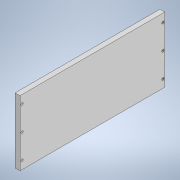
# Autodesk Inventor part: cab_L_L
Saved by Autodesk Inventor 2022 (Build 260153000, 153)
## iProperties
Created: 2023-03-05
Part Number: cab_L_L
Material: Generic
Document SubType Name: Modeling
Designer: Bunny
Density: 1 g/cm^3
Appearance: Default
Author: Bunny
Autodesk Inventor part; units mm, degrees
ref_plane "YZ Plane" through (0, 0, 0) normal (1, 0, 0) x (0, 1, 0)
ref_plane "XZ Plane" through (0, 0, 0) normal (0, 1, 0) x (-1, 0, 0)
ref_plane "XY Plane" through (0, 0, 0) normal (0, 0, 1) x (1, 0, 0)
sketch "Sketch1" plane through (0, 0, 0) normal (1, 0, 0) x (0, 1, 0)
  line L0 (-52.1082, -123.2649) -> (27.8918, -123.2649)
  line L1 (27.8918, -123.2649) -> (27.8918, 54.7351)
  line L2 (27.8918, 54.7351) -> (-52.1082, 54.7351)
  line L3 (-52.1082, 54.7351) -> (-52.1082, -123.2649)
  point P0 (0, 0)
  dimension "d0" = 178
  dimension "d1" = 80
  constraints: 8 end point, 2 parallel, 1 horizontal, 1 perpendicular
  measures "d0" distance of L0.end L1.end
  measures "d1" distance of L1.end L2.end
extrude "Extrusion1" add sketch "Sketch1" along normal blind 6
sketch "Sketch2" plane through (6, 0, 0) normal (1, 0, 0) x (0, 0, -1)
  circle A0 centre (-52.2351, 17.8918) radius 1.405
  line L0 (-54.7351, 27.8918) -> (-54.7351, -52.1082) projected
  line L1 (123.2649, 27.8918) -> (-54.7351, 27.8918) projected
  point P0 (0, 0)
  dimension "d4" = 2.81
  dimension "d5" = 2.5
  dimension "d6" = 10
  constraints: 1 centre point
  measures "d4" diameter of A0
  measures "d5" distance from line of L0 A0.centre
  measures "d6" distance from line of L1 A0.centre
extrude "Extrusion2" cut sketch "Sketch2" against normal blind 10
pattern_linear "Rectangular Pattern1" count 3 spacing 30 along (0, -1, 0) count 2 spacing -173 along (0, 0, 1) of "Extrusion2"
equation "\"d0\" = -2 * CornerOffset + BoxWidth - 2 * SheetThickness"
equation "\"d1\" = BoxHeight"
equation "\"d2\" = SheetThickness"
equation "\"d4\" = M3Hole"
equation "\"d5\" = HoleOffset"
equation "\"BoxHeight\" = 80"
equation "\"SheetThickness\" = 6"
equation "\"CornerOffset\" = 5"
equation "\"M3Hole\" = 2.81"
equation "\"HoleOffset\" = 2.5"
equation "\"BoxWidth\" = 200"
body "Solid1"
